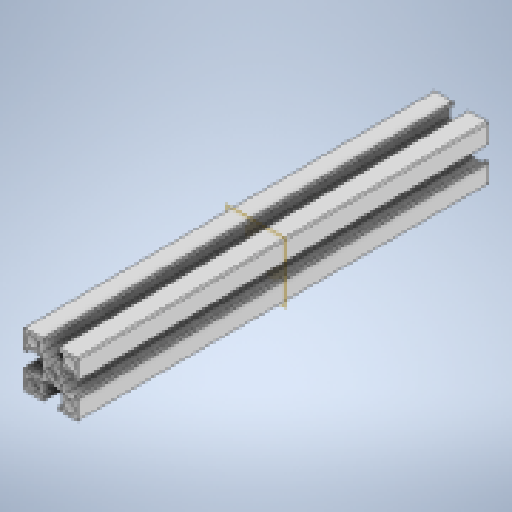
# Autodesk Inventor part: Aluminum_Profile_2020
Saved by Autodesk Inventor 2024.2 (Build 282272000, 272)
## iProperties
Created: 2023-12-13
Part Number: Aluminum_Profile_2020
Material: Generic
Document SubType Name: Modeling
Designer: 박동준
Density: 1 g/cm^3
Appearance: Default
Author: 박동준
Autodesk Inventor part; units mm, degrees
ref_plane "YZ Plane" through (0, 0, 0) normal (1, 0, 0) x (0, 1, 0)
ref_plane "XZ Plane" through (0, 0, 0) normal (0, 1, 0) x (-1, 0, 0)
ref_plane "XY Plane" through (0, 0, 0) normal (0, 0, 1) x (1, 0, 0)
sketch "Sketch1" plane through (0, 0, 0) normal (0, 0, 1) x (1, 0, 0)
  line L0 (0, 0) -> (12.2143, 12.2143) construction
  line L1 (0, 0) -> (10, 0) construction
  circle A0 centre (0, 0) radius 2.15
  circle A1 centre (7, 7) radius 2
  circle A2 centre (-7, 7) radius 2
  circle A3 centre (-7, -7) radius 2
  circle A4 centre (7, -7) radius 2
  line L2 (2.95, 10) -> (9.5, 10)
  line L3 (10, 9.5) -> (10, 2.95)
  line L4 (9.7, 2.65) -> (8.9, 2.65)
  line L5 (8.6, 2.95) -> (8.6, 4.2)
  line L6 (4.2, 4.4357) -> (4.2, 8.6)
  line L7 (2.65, 9.7) -> (2.65, 8.9)
  line L8 (2.95, 8.6) -> (4.2, 8.6)
  line L9 (0, 14.2934) -> (0, -14.2934) construction
  arc A5 (2.95, 10) -> (2.65, 9.7) centre (2.95, 9.7) ccw
  arc A6 (2.65, 8.9) -> (2.95, 8.6) centre (2.95, 8.9) ccw
  arc A7 (8.6, 2.95) -> (8.9, 2.65) centre (8.9, 2.95) ccw
  arc A8 (9.7, 2.65) -> (10, 2.95) centre (9.7, 2.95) ccw
  arc A9 (10, 9.5) -> (9.5, 10) centre (9.5, 9.5) ccw
  circle A10 centre (0, 7.1516) radius 5.0016 construction
  circle A11 centre (7.1516, 0) radius 5.0016 construction
  line L10 (8.6, 4.2) -> (4.4357, 4.2)
  line L11 (0, 3) -> (1.9054, 3.3)
  arc A12 (1.9054, 3.3) -> (4.2, 4.4357) centre (0, 10.0357) ccw
  line L12 (3, 0) -> (3.3, 1.9054)
  arc A13 (4.4357, 4.2) -> (3.3, 1.9054) centre (10.0357, 0) ccw
  line L13 (-3, 0) -> (-3.3, 1.9054)
  arc A14 (-3.3, 1.9054) -> (-4.4357, 4.2) centre (-10.0357, 0) ccw
  arc A15 (-4.2, 4.4357) -> (-1.9054, 3.3) centre (0, 10.0357) ccw
  line L14 (0, 3) -> (-1.9054, 3.3)
  line L15 (-4.4357, 4.2) -> (-8.6, 4.2)
  line L16 (-8.6, 2.95) -> (-8.6, 4.2)
  arc A16 (-8.9, 2.65) -> (-8.6, 2.95) centre (-8.9, 2.95) ccw
  line L17 (-9.7, 2.65) -> (-8.9, 2.65)
  arc A17 (-10, 2.95) -> (-9.7, 2.65) centre (-9.7, 2.95) ccw
  line L18 (-10, 2.95) -> (-10, 9.5)
  arc A18 (-9.5, 10) -> (-10, 9.5) centre (-9.5, 9.5) ccw
  line L19 (-9.5, 10) -> (-2.95, 10)
  line L20 (-4.2, 8.6) -> (-4.2, 4.4357)
  line L21 (-2.95, 8.6) -> (-4.2, 8.6)
  arc A19 (-2.95, 8.6) -> (-2.65, 8.9) centre (-2.95, 8.9) ccw
  line L22 (-2.65, 9.7) -> (-2.65, 8.9)
  arc A20 (-2.65, 9.7) -> (-2.95, 10) centre (-2.95, 9.7) ccw
  line L23 (0, -3) -> (-1.9054, -3.3)
  arc A21 (-1.9054, -3.3) -> (-4.2, -4.4357) centre (0, -10.0357) ccw
  arc A22 (-4.4357, -4.2) -> (-3.3, -1.9054) centre (-10.0357, 0) ccw
  line L24 (-3, 0) -> (-3.3, -1.9054)
  line L25 (-4.2, -4.4357) -> (-4.2, -8.6)
  line L26 (-2.95, -8.6) -> (-4.2, -8.6)
  arc A23 (-2.65, -8.9) -> (-2.95, -8.6) centre (-2.95, -8.9) ccw
  line L27 (-2.65, -9.7) -> (-2.65, -8.9)
  arc A24 (-2.95, -10) -> (-2.65, -9.7) centre (-2.95, -9.7) ccw
  line L28 (-2.95, -10) -> (-9.5, -10)
  arc A25 (-10, -9.5) -> (-9.5, -10) centre (-9.5, -9.5) ccw
  line L29 (-10, -9.5) -> (-10, -2.95)
  line L30 (-8.6, -4.2) -> (-4.4357, -4.2)
  line L31 (-8.6, -2.95) -> (-8.6, -4.2)
  arc A26 (-8.6, -2.95) -> (-8.9, -2.65) centre (-8.9, -2.95) ccw
  line L32 (-9.7, -2.65) -> (-8.9, -2.65)
  arc A27 (-9.7, -2.65) -> (-10, -2.95) centre (-9.7, -2.95) ccw
  line L33 (3, 0) -> (3.3, -1.9054)
  arc A28 (3.3, -1.9054) -> (4.4357, -4.2) centre (10.0357, 0) ccw
  arc A29 (4.2, -4.4357) -> (1.9054, -3.3) centre (0, -10.0357) ccw
  line L34 (0, -3) -> (1.9054, -3.3)
  line L35 (4.4357, -4.2) -> (8.6, -4.2)
  line L36 (8.6, -2.95) -> (8.6, -4.2)
  arc A30 (8.9, -2.65) -> (8.6, -2.95) centre (8.9, -2.95) ccw
  line L37 (9.7, -2.65) -> (8.9, -2.65)
  arc A31 (10, -2.95) -> (9.7, -2.65) centre (9.7, -2.95) ccw
  line L38 (10, -2.95) -> (10, -9.5)
  arc A32 (9.5, -10) -> (10, -9.5) centre (9.5, -9.5) ccw
  line L39 (9.5, -10) -> (2.95, -10)
  line L40 (4.2, -8.6) -> (4.2, -4.4357)
  line L41 (2.95, -8.6) -> (4.2, -8.6)
  arc A33 (2.95, -8.6) -> (2.65, -8.9) centre (2.95, -8.9) ccw
  line L42 (2.65, -9.7) -> (2.65, -8.9)
  arc A34 (2.65, -9.7) -> (2.95, -10) centre (2.95, -9.7) ccw
  point P0 (10, 2.65)
  point P1 (8.6, 2.65)
  point P2 (-2.65, 10)
  point P3 (-2.65, 8.6)
  point P4 (-10, -2.65)
  point P5 (-8.6, -2.65)
  point P6 (2.65, -10)
  point P7 (2.65, -8.6)
  dimension "d1" = 45
  dimension "d2" = 4.3
  dimension "d3" = 4
  dimension "d6" = 360
  dimension "d9" = 2.65
  dimension "d10" = 4.2
  dimension "d11" = 1.4
  dimension "d12" = 7
  dimension "d13" = 10
  dimension "d14" = 10
  dimension "d15" = 1.4
  dimension "d16" = 2.65
  dimension "d18" = 0.3
  dimension "d19" = 0.5
  dimension "d22" = 4.2
  dimension "d24" = 6.7
  dimension "d25" = 0.3
  dimension "d26" = 7
  dimension "d27" = 6.7
  dimension "d28" = 0.3
  dimension "d29" = 7
  dimension "d32" = 360
  constraints: 86 end point, 56 point on circle, 33 centre point, 20 point on line, 10 tangent, 4 perpendicular, 3 coincident, 3 equal radius, 3 horizontal, 2 vertical, 2 vertical alignment, 1 horizontal alignment, 1 midpoint, 1 symmetric about line, 195 other
  measures "d1" angle of L1 L0
  measures "d2" diameter of A0
  measures "d3" diameter of A1
  measures "d9" distance between parallel lines of L7 L9
  measures "d10" distance between parallel lines of L9 L6
  measures "d11" distance between parallel lines of L8 L2
  measures "d12" distance from line of L9 A1.centre
  measures "d13" distance between parallel lines of L9 L3
  measures "d14" distance from line of L2 L0.start
  measures "d15" distance of point (10, 2.65) point (8.6, 2.65)
  measures "d16" distance between parallel lines of L1 L4
  measures "d18" radius of A5
  measures "d19" radius of A9
  measures "d22" distance between parallel lines of L1 L10
  measures "d24" distance from line of L2 L11.end
  measures "d25" vertical distance of L11.end L11.start
  measures "d26" radius of A12
  measures "d27" distance from line of L3 L12.end
  measures "d28" horizontal distance of L12.end L12.start
  measures "d29" radius of A13
extrude "Extrusion1" add sketch "Sketch1" along normal blind 150
sketch "Sketch2" plane through (2.95, 10, 150) normal (0, 1, 0) x (1, 0, 0)
  line L0 (-2.95, 150) -> (-2.95, 0) projected
  circle A0 centre (-2.95, 6) radius 2.15
  dimension "d36" = 4.3
  dimension "d37" = 6
  constraints: 1 centre point, 1 point on line
  measures "d36" diameter of A0
  measures "d37" distance of A0.centre L0.end
extrude "Extrusion2" cut sketch "Sketch2" against normal blind 10
ref_plane "Work Plane1" through (0, 0, 75) normal (0, 0, 1) x (1, 0, 0)
body "Solid1"
